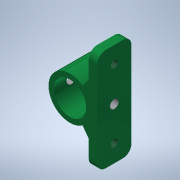
# Autodesk Inventor part: Mancal_Fixo
Saved by Autodesk Inventor 2022 (Build 260153000, 153)
## iProperties
Created: 2016-02-21
Part Number: Mancal_Fixo
Material: Genérico
Document SubType Name: Modeling
Designer: Everton
Density: 1 g/cm^3
Appearance: Padrão
Author: Everton
Autodesk Inventor part; units mm, degrees
ref_plane "YZ Plane" through (0, 0, 0) normal (1, 0, 0) x (0, 1, 0)
ref_plane "XZ Plane" through (0, 0, 0) normal (0, 1, 0) x (-1, 0, 0)
ref_plane "XY Plane" through (0, 0, 0) normal (0, 0, 1) x (1, 0, 0)
sketch "Sketch1" plane through (0, 0, 0) normal (0, 1, 0) x (-1, 0, 0)
  arc A0 (1.1623, -30.2706) -> (1.1135, 10.0138) centre (15.9463, -10.1104) ccw
  circle A1 centre (15.9463, -10.1104) radius 19
  line L0 (-9.0537, -10.1104) -> (-6.0537, -10.1104)
  line L1 (-6.0537, -10.1104) -> (-6.0537, 49.8896)
  line L2 (-6.0537, 49.8896) -> (-16.0537, 49.8896)
  line L3 (-16.0537, 49.8896) -> (-16.0537, -70.1104)
  line L4 (-16.0537, -70.1104) -> (-6.0537, -70.1104)
  line L5 (-6.0537, -70.1104) -> (-6.0537, -10.1104)
  line L6 (-6.0537, 19.8896) -> (1.1135, 10.0138)
  line L7 (15.9463, -10.1104) -> (15.8318, -10.2667)
  line L8 (1.1623, -30.2706) -> (-6.0537, -40.1104)
  point P0 (0, 0)
  dimension "d0" = 50
  dimension "d1" = 38
  dimension "d2" = 3
  dimension "d4" = 10
  dimension "d5" = 120
  dimension "d11" = 0
  constraints: 18 end point, 5 perpendicular, 2 centre point, 2 midpoint, 2 point on circle, 1 coincident, 1 horizontal, 1 point on line
  measures "d0" diameter of A0
  measures "d1" diameter of A1
  measures "d2" distance of L0.start L0.end
  measures "d4" distance of L1.end L2.end
  measures "d5" distance of L2.end L3.end
  measures "d11" distance from line of L0 A0.centre
extrude "Extrusion1" add sketch "Sketch1" along normal blind 40
sketch "Sketch2" plane through (16.0537, 0, 49.8896) normal (1, 0, 0) x (0, 0, -1)
  line L0 (0, 0) -> (0, 40) projected
  line L1 (0, 20) -> (120, 20)
  line L2 (120, 0) -> (120, 40) projected
  circle A0 centre (60, 20) radius 5
  circle A1 centre (20, 20) radius 4
  circle A2 centre (100, 20) radius 4
  point P0 (49.8896, 0)
  dimension "d14" = 10
  dimension "d15" = 8
  dimension "d16" = 8
  dimension "d17" = 20
  dimension "d18" = 20
  constraints: 3 centre point, 3 midpoint, 2 end point, 2 point on line
  measures "d14" diameter of A0
  measures "d15" diameter of A1
  measures "d16" diameter of A2
  measures "d17" distance of L1.end A2.centre
  measures "d18" distance of L1.start A1.centre
hole "Hole1" at (16.0537, 20, 29.8896) at (16.0537, 20, -50.1104) direction (-1, 0, 0) diameter 8.376 depth 27.3 tip angle 118 thread size "M10x1.5" class "6H" standard "ISO Metric profile"
fillet "Fillet1" radius 10 4 edges at (11.0537, 40, 49.8896) (11.0537, 0, 49.8896) (11.0537, 40, -70.1104) (11.0537, 0, -70.1104)
extrude "Extrusion2" cut sketch "Sketch2" against normal blind 100 contours A0 L1 | L1 A0
body "Solid1"
